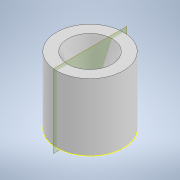
# Autodesk Inventor part: ptfe_catch_no_mount
Saved by Autodesk Inventor 2020 (Build 240168000, 168)
## iProperties
Created: 2021-06-26
Part Number: ptfe_catch_no_mount
Material: Generic
Document SubType Name: Modeling
Designer: pab2
Density: 1 g/cm^3
Appearance: Default
Author: pab2
Autodesk Inventor part; units mm, degrees
ref_plane "YZ Plane" through (0, 0, 0) normal (1, 0, 0) x (0, 1, 0)
ref_plane "XZ Plane" through (0, 0, 0) normal (0, 1, 0) x (-1, 0, 0)
ref_plane "XY Plane" through (0, 0, 0) normal (0, 0, 1) x (1, 0, 0)
sketch "Sketch1" plane through (0, 0, 0) normal (1, 0, 0) x (0, 1, 0)
  line L0 (0, 0) -> (38.1, 0)
  line L1 (38.1, 0) -> (38.1, -19.05)
  line L2 (38.1, -19.05) -> (0, -19.05)
  line L3 (0, -19.05) -> (0, 0)
  line L4 (0, 0) -> (0, -0.7937)
  line L5 (0, -0.7937) -> (12.7, -0.7937)
  line L6 (12.7, -0.7937) -> (38.1, -12.638) construction
  line L7 (38.1, -12.638) -> (38.1, 0)
  line L8 (0, 0) -> (0, -0.7937)
  line L9 (12.7, -0.7937) -> (38.1, -12.638)
  line L10 (12.7, -0.7937) -> (40.7258, -0.7937) construction
  line L11 (0, -19.05) -> (5.8372, -13.2128)
  line L12 (0, -19.05) -> (8.255, -19.05) construction
  point P0 (8.255, 8.255)
  dimension "partH" = 38.1
  dimension "partR" = 19.05
  dimension "tubeID" = 0.7937
  dimension "straightDepth" = 12.7
  dimension "funnelTaperAngle" = 155
  dimension "taperAngle" = 25
  dimension "d15" = 8.255
  dimension "d16" = 45
  constraints: 26 end point, 3 horizontal, 3 parallel, 2 coincident, 2 equal length, 2 perpendicular, 2 point on line, 1 collinear
  measures "partH" distance of L1.end L2.end
  measures "partR" distance of L0.end L1.end
  measures "tubeID" distance of L0.start L4.end
  measures "straightDepth" distance of L4.end L5.end
  measures "funnelTaperAngle" angle of L5 L6
  measures "taperAngle" angle of L9 L10
  measures "d15" distance of L11.start L11.end
  measures "d16" angle of L12 L11
revolve "Revolution1" add sketch "Sketch1" angle 360 about axis through (0, 0, 0) along (0, 1, 0) contours L5 L9 L1 L2 L3
sketch "Sketch2" plane through (0, 0, 0) normal (0, -1, 0) x (1, 0, 0)
  point P0 (0, 0)
  point P1 (0, 0)
  constraints: 1 coincident
hole "Hole1" at (0, 0, 0) direction (0, 1, 0) diameter 5.3594 depth 9.525 tip angle 118 thread size "1/4-28 UNF" class "2B" standard "ANSI Unified Screw Threads"
sketch "Sketch3" plane through (0, 0, 0) normal (0, -1, 0) x (1, 0, 0)
  circle A0 centre (0, 0) radius 0.7937 projected
  line L0 (0, 0) -> (0, -19.05)
  circle A1 centre (0, 0) radius 19.05 projected
  constraints: 2 end point, 1 vertical, 1 vertical alignment, 1 other
ref_plane "Work Plane1" through (0, 0, 0) normal (-1, 0, 0) x (0, 0, -1)
sketch "Sketch4" plane through (0, 0, 0) normal (-1, 0, 0) x (0, 0, -1)
  line L0 (19.05, 0) -> (-19.05, 0) projected
  line L1 (-19.05, 0) -> (-11.8658, -7.1842)
  line L2 (-19.05, 0) -> (-8.89, 0) construction
  line L3 (19.05, 0) -> (11.8658, -7.1842)
  line L4 (19.05, 0) -> (29.21, 0) construction
  point P0 (0, 0)
  dimension "d18" = 10.16
  dimension "d19" = 45
  dimension "d20" = 10.16
  dimension "d21" = 135
  constraints: 8 end point, 2 equal length, 2 horizontal
  measures "d18" distance of L0.end L1.end
  measures "d19" angle of L1 L2
  measures "d20" distance of L0.start L3.end
  measures "d21" angle of L3 L4
body "Solid1"
